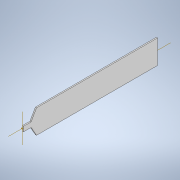
# Autodesk Inventor part: 2DBoquilla0.4
Saved by Autodesk Inventor 2022 (Build 260153000, 153)
## iProperties
Created: 2022-04-01
Part Number: 2DBoquilla0.4
Material: Genérico
Document SubType Name: Modeling
Designer: anuar
Density: 1 g/cm^3
Appearance: Valor por defecto
Author: anuar
Autodesk Inventor part; units mm, degrees
ref_plane "YZ Plane" through (0, 0, 0) normal (1, 0, 0) x (0, 1, 0)
ref_plane "XZ Plane" through (0, 0, 0) normal (0, 1, 0) x (-1, 0, 0)
ref_plane "XY Plane" through (0, 0, 0) normal (0, 0, 1) x (1, 0, 0)
sketch "Boceto2" plane through (0, 0, 0) normal (1, 0, 0) x (0, 1, 0)
  line L0 (-0.2, 0) -> (-0.2, -0.62)
  line L1 (-0.2, -0.62) -> (-0.99, -1.0761)
  line L2 (-0.99, -1.0761) -> (-0.99, -11.1361)
  line L3 (-0.99, -11.1361) -> (0, -11.1361)
  line L4 (0, 0) -> (-0.2, 0)
  line L5 (0, -11.1361) -> (0, 0)
  dimension "d10" = 0.2
  dimension "d11" = 0.62
  dimension "d12" = 10.06
  dimension "d13" = 60
  dimension "d14" = 0.99
  constraints: 12 end point, 1 parallel
  measures "d10" distance from line of L4.start L0
  measures "d11" distance of L0.start L0.end
  measures "d12" distance of L1.end L2.end
  measures "d13" angle of L5 L1
  measures "d14" distance between parallel lines of L5 L2
extrude "Extrusión1" add sketch "Boceto2" along normal blind 0.1
mirror "Simetría1" about plane through (0, 0, -11.1361) normal (0, 1, 0) of "Extrusión1"
equation "\"d10\" = 0.5 * d18"
equation "\"d11\" = d15"
equation "\"d12\" = d16"
equation "\"d13\" = d17"
equation "\"d14\" = 0.5 * d19"
equation "\"Dc\" = 0.4"
equation "\"Lc\" = 0.62"
equation "\"Ln\" = 10.06"
equation "\"Do\" = 1.98"
equation "\"alfa\" = 60deg"
equation "\"d15\" = 0.62"
equation "\"d16\" = 10.06"
equation "\"d17\" = 60deg"
equation "\"d18\" = 0.4"
equation "\"d19\" = 1.98"
